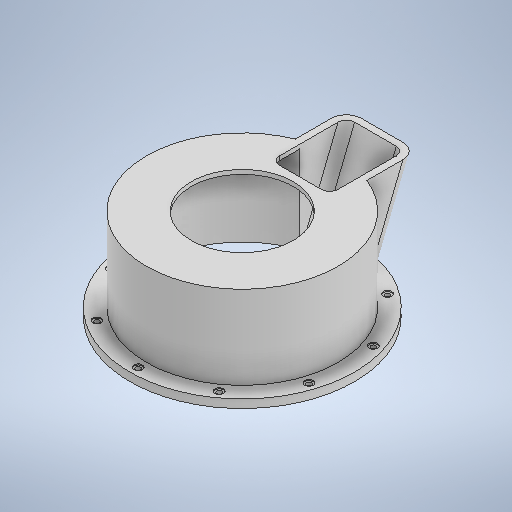
# Autodesk Inventor part: Vibrometer Housing
Saved by Autodesk Inventor 2026.2 (Build 302298000, 298)
## iProperties
Created: 2026-03-24
Part Number: Vibrometer Housing
Material: Generic
Document SubType Name: Modeling
Designer: mumin
Density: 1 g/cm^3
Appearance: Default
Author: mumin
Autodesk Inventor part; units mm, degrees
ref_plane "YZ Plane" through (0, 0, 0) normal (1, 0, 0) x (0, 1, 0)
ref_plane "XZ Plane" through (0, 0, 0) normal (0, 1, 0) x (-1, 0, 0)
ref_plane "XY Plane" through (0, 0, 0) normal (0, 0, 1) x (1, 0, 0)
sketch "Sketch1" plane through (0, 0, 0) normal (1, 0, 0) x (0, 1, 0)
  line L0 (0, 0) -> (120, 0)
  line L1 (110, -61.25) -> (105, -61.25)
  line L2 (105, -61.25) -> (105, -110)
  line L3 (105, -110) -> (0, -110)
  line L4 (0, -110) -> (0, -135)
  line L5 (0, -135) -> (10, -135)
  line L6 (10, -135) -> (10, -115)
  line L7 (10, -115) -> (110, -115)
  line L8 (110, -115) -> (110, -61.25)
  line L9 (0, -114) -> (2, -114)
  line L10 (2, -114) -> (2, -117)
  line L11 (2, -117) -> (0, -117)
  line L12 (0, -117) -> (0, -114)
  point P0 (2, -115)
  point P1 (1, -114)
  dimension "d1" = 270
  dimension "d2" = 220
  dimension "d3" = 230
  dimension "d4" = 122.5
  dimension "d5" = 10
  dimension "d6" = 5
  dimension "d7" = 110
  dimension "d21" = 228
  dimension "d22" = 3
  dimension "d24" = 2
  constraints: 26 end point, 8 perpendicular, 3 horizontal, 2 parallel, 2 point on line
  measures "d1" diameter of L5 L0
  measures "d2" diameter of L3 L0
  measures "d3" diameter of L7 L0
  measures "d4" diameter of L1 L0
  measures "d5" distance between parallel lines of L4 L6
  measures "d6" distance between parallel lines of L2 L8
  measures "d7" distance between parallel lines of L4 L8
  measures "d21" diameter of L9 L0
  measures "d22" distance of L9.end L10.end
  measures "d24" distance from line of L4 L10.end
revolve "Base Cylinder" add sketch "Sketch1" angle 360 about axis through (0, 0, 0) along (0, 1, 0)
sketch "Sketch2" plane through (0, 10, 0) normal (0, 1, 0) x (1, 0, 0)
  point P0 (0, 0)
  point P1 (0, 125)
  point P2 (-73.4732, 101.1271)
  point P3 (-118.8821, 38.6271)
  point P4 (-118.8821, -38.6271)
  point P5 (-73.4732, -101.1271)
  point P6 (0, -125)
  point P7 (73.4732, -101.1271)
  point P8 (118.8821, -38.6271)
  point P9 (118.8821, 38.6271)
  point P10 (73.4732, 101.1271)
  dimension "d9" = 125
  dimension "d12" = 360
  constraints: 11 other
  measures "d9" distance of point (0, 0) point (0, 125)
hole "M5 Mounting Holes" at (0, 10, -125) at (-73.4732, 10, -101.1271) at (-118.8821, 10, -38.6271) at (-118.8821, 10, 38.6271) at (-73.4732, 10, 101.1271) at (0, 10, 125) at (73.4732, 10, 101.1271) at (118.8821, 10, 38.6271) at (118.8821, 10, -38.6271) at (73.4732, 10, -101.1271) direction (0, -1, 0) diameter 5.9 end through all counterbore diameter 10.2 counterbore depth 1.2
sketch "Sketch3" plane through (0, 110, 0) normal (0, 1, 0) x (1, 0, 0)
  line L0 (0, 143.2495) -> (0, 0)
  circle A0 centre (0, 0) radius 61.25 projected
  circle A1 centre (0, 0) radius 115 projected
  line L1 (-35, 109.5445) -> (-35, 80)
  line L2 (0, 70) -> (-25, 70)
  arc A2 (-35, 80) -> (-25, 70) centre (-25, 80) ccw
  line L3 (35, 109.5445) -> (35, 80)
  line L4 (0, 70) -> (25, 70)
  arc A3 (25, 70) -> (35, 80) centre (25, 80) ccw
  dimension "d25" = 10
  dimension "d26" = 70
  dimension "d27" = 70
  constraints: 10 end point, 4 point on circle, 4 symmetric about line, 2 centre point, 2 tangent, 2 vertical, 1 perpendicular, 1 point on line, 3 other
  measures "d25" radius of A2
  measures "d26" diameter of L1 L0
  measures "d27" distance from line of L0.end L2
extrude "Access Cutout" cut sketch "Sketch3" against normal up to surface (100 mm away) contours A1 L3 A3 L4 L0 | L0 L2 A2 L1 A1
sketch "Sketch4" plane through (0, 110, 0) normal (0, 1, 0) x (1, 0, 0)
  line L0 (35, 109.5445) -> (35, 80) projected
  arc A0 (25, 70) -> (35, 80) centre (25, 80) ccw projected
  line L1 (25, 70) -> (-25, 70) projected
  arc A1 (-35, 80) -> (-25, 70) centre (-25, 80) ccw projected
  line L2 (-35, 80) -> (-35, 109.5445) projected
  arc A2 (-35, 109.5445) -> (35, 109.5445) centre (0, 0) ccw projected
  circle A3 centre (0, 0) radius 61.25 projected
  line L3 (0, 0) -> (0, 180)
  line L4 (-35, 109.5445) -> (-35, 150)
  line L5 (-25, 160) -> (0, 160)
  arc A4 (-25, 160) -> (-35, 150) centre (-25, 150) ccw
  line L6 (0, 168) -> (-25, 168)
  arc A5 (-25, 168) -> (-43, 150) centre (-25, 150) ccw
  line L7 (-43, 150) -> (-43, 106.6583)
  line L8 (35, 109.5445) -> (35, 150)
  line L9 (25, 160) -> (0, 160)
  arc A6 (35, 150) -> (25, 160) centre (25, 150) ccw
  line L10 (0, 168) -> (25, 168)
  arc A7 (43, 150) -> (25, 168) centre (25, 150) ccw
  line L11 (43, 150) -> (43, 106.6583)
  dimension "d31" = 10
  dimension "d32" = 8
  dimension "d33" = 160
  constraints: 18 end point, 9 point on circle, 6 symmetric about line, 4 centre point, 2 tangent, 2 vertical, 1 parallel, 1 perpendicular, 1 point on line, 3 other
  measures "d31" radius of A4
  measures "d32" distance between parallel lines of L5 L6
  measures "d33" distance from line of point (0, 0) L5
sketch "Sketch5" plane through (0, 0, 0) normal (1, 0, 0) x (0, 1, 0)
  line L0 (10, -96.0271) -> (10, -106.2271) projected
  line L1 (10, -33.5271) -> (10, -43.7271) projected
  line L2 (10, 43.7271) -> (10, 33.5271) projected
  line L3 (10, 106.2271) -> (10, 96.0271) projected
  line L4 (10, 130.1) -> (10, 119.9) projected
  line L5 (10, 106.2271) -> (10, 96.0271) projected
  line L6 (10, 43.7271) -> (10, 33.5271) projected
  line L7 (10, -33.5271) -> (10, -43.7271) projected
  line L8 (10, -96.0271) -> (10, -106.2271) projected
  line L9 (10, -119.9) -> (10, -130.1) projected
  line L10 (10, -109.5445) -> (10, -109.5445) projected
  line L11 (10, -104.2833) -> (10, -109.5445) projected
  line L12 (10, -104.2833) -> (10, -104.2833) projected
  line L13 (10, -109.5445) -> (10, -104.2833) projected
  line L14 (10, -135) -> (10, 135) projected
  line L15 (110, -168) -> (10, -127.5974)
  point P0 (0, 0)
  dimension "d34" = 68
  constraints: 2 end point, 1 point on line
  measures "d34" angle of L14 L15
sweep "Angle Bracket" add profiles "Sketch4" path "Sketch5" keep normal constant yes path curves L15 contours L8 A6 L9 L3 L10 A7 L11 A2 | L7 A5 L6 L3 L5 A4 L4 A2
sketch "Sketch6" plane through (0, 105, 0) normal (0, -1, 0) x (1, 0, 0)
  line L0 (35, -80) -> (35, -104.2833) projected
  arc A0 (35, -104.2833) -> (-35, -104.2833) centre (0, 0) ccw projected
  line L1 (-35, -104.2833) -> (-35, -80) projected
  arc A1 (-25, -70) -> (-35, -80) centre (-25, -80) ccw projected
  line L2 (-25, -70) -> (25, -70) projected
  arc A2 (35, -80) -> (25, -70) centre (25, -80) ccw projected
  circle A3 centre (0, 0) radius 61.25 projected
extrude "Remove Sweep Excess" cut sketch "Sketch6" along normal up to surface (105 mm away)
body "Solid1"
